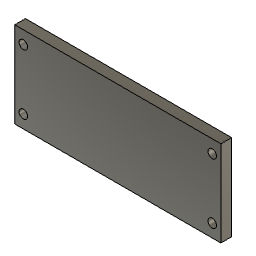
cementform_Wmiddle_80x40_plateB (Autodesk Fusion 360 design; units mm, degrees)
Autodesk Fusion 360 part; units mm, degrees
sketch "baseplate" plane through (0, 0, 0) normal (0, 1, 0) x (1, 0, 0)
  line L0 (0, 0) -> (80, 0)
  line L1 (80, 0) -> (80, -40)
  line L2 (80, -40) -> (0, -40)
  line L3 (0, -40) -> (0, 0)
  dimension "d1" = 80
  dimension "d2" = 40
  constraint horizontal L0
  constraint vertical L1
  constraint horizontal L2
  constraint vertical L3
  constraint coincident L0.start L3.end
  measures "d1" distance of L0.start L0.end
  measures "d2" distance of L0.start L2.end
sketch "pryamid_base" plane through (0, 0, 0) normal (0, 1, 0) x (1, 0, 0)
  line L0 (5, -35) -> (15, -35)
  line L1 (15, -35) -> (15, -25)
  line L2 (15, -25) -> (5, -25)
  line L3 (5, -25) -> (5, -35)
  line L4 (35, -35) -> (35, -25)
  line L5 (35, -25) -> (25, -25)
  line L6 (25, -35) -> (35, -35)
  line L7 (25, -25) -> (25, -35)
  line L8 (75, -35) -> (75, -25)
  line L9 (45, -35) -> (55, -35)
  line L10 (55, -25) -> (45, -25)
  line L11 (65, -25) -> (65, -35)
  line L12 (65, -35) -> (75, -35)
  line L13 (55, -35) -> (55, -25)
  line L14 (45, -25) -> (45, -35)
  line L15 (75, -25) -> (65, -25)
  line L16 (35, -5) -> (25, -5)
  line L17 (35, -15) -> (35, -5)
  line L18 (15, -5) -> (5, -5)
  line L19 (25, -5) -> (25, -15)
  line L20 (45, -15) -> (55, -15)
  line L21 (55, -15) -> (55, -5)
  line L22 (5, -5) -> (5, -15)
  line L23 (45, -5) -> (45, -15)
  line L24 (75, -15) -> (75, -5)
  line L25 (65, -5) -> (65, -15)
  line L26 (75, -5) -> (65, -5)
  line L27 (55, -5) -> (45, -5)
  line L28 (65, -15) -> (75, -15)
  line L29 (5, -15) -> (15, -15)
  line L30 (15, -15) -> (15, -5)
  line L31 (25, -15) -> (35, -15)
  dimension "d3" = 10
  dimension "d4" = 10
  dimension "d5" = 10
  dimension "d6" = 10
  dimension "d7" = 10
  dimension "d8" = 10
  dimension "d9" = 10
  dimension "d10" = 10
  dimension "d11" = 10
  dimension "d12" = 10
  dimension "d13" = 10
  dimension "d14" = 10
  dimension "d15" = 10
  dimension "d16" = 10
  dimension "d17" = 10
  dimension "d18" = 10
  constraint horizontal L0
  constraint vertical L1
  constraint horizontal L2
  constraint vertical L3
  constraint horizontal L6
  constraint vertical L4
  constraint horizontal L5
  constraint vertical L7
  constraint horizontal L9
  constraint vertical L13
  constraint horizontal L10
  constraint vertical L14
  constraint horizontal L12
  constraint vertical L8
  constraint horizontal L15
  constraint vertical L11
  constraint horizontal L29
  constraint vertical L30
  constraint horizontal L18
  constraint vertical L22
  constraint horizontal L31
  constraint vertical L17
  constraint horizontal L16
  constraint vertical L19
  constraint horizontal L20
  constraint vertical L21
  constraint horizontal L27
  constraint vertical L23
  constraint horizontal L28
  constraint vertical L24
  constraint horizontal L26
  constraint vertical L25
  measures "d3" distance of L0.start L0.end
  measures "d4" distance of L0.start L2.end
  measures "d5" distance of L6.start L4.start
  measures "d6" distance of L6.start L5.end
  measures "d7" distance of L9.start L9.end
  measures "d8" distance of L9.start L10.end
  measures "d9" distance of L8.start L11.end
  measures "d10" distance of L11.start L11.end
  measures "d11" distance of L22.end L29.end
  measures "d12" distance of L22.end L18.end
  measures "d13" distance of L17.start L19.end
  measures "d14" distance of L16.end L19.end
  measures "d15" distance of L20.start L20.end
  measures "d16" distance of L20.start L23.start
  measures "d17" distance of L24.start L25.end
  measures "d18" distance of L25.start L25.end
ref_plane "WorkPlane1" through (0, 4.5, 0) normal (0, 1, 0) x (0, 0, 1)
sketch "pryamid_offsetplane" plane through (0, 4.5, 0) normal (0, 1, 0) x (1, 0, 0)
  line L0 (7.5, -32.5) -> (12.5, -32.5)
  line L1 (12.5, -32.5) -> (12.5, -27.5)
  line L2 (12.5, -27.5) -> (7.5, -27.5)
  line L3 (7.5, -27.5) -> (7.5, -32.5)
  line L4 (27.5, -27.5) -> (27.5, -32.5)
  line L5 (32.5, -32.5) -> (32.5, -27.5)
  line L6 (27.5, -32.5) -> (32.5, -32.5)
  line L7 (32.5, -27.5) -> (27.5, -27.5)
  line L8 (7.5, -27.5) -> (7.5, -32.5)
  line L9 (12.5, -32.5) -> (12.5, -27.5)
  line L10 (7.5, -32.5) -> (12.5, -32.5)
  line L11 (12.5, -27.5) -> (7.5, -27.5)
  line L12 (47.5, -27.5) -> (47.5, -32.5)
  line L13 (52.5, -32.5) -> (52.5, -27.5)
  line L14 (47.5, -32.5) -> (52.5, -32.5)
  line L15 (52.5, -27.5) -> (47.5, -27.5)
  line L16 (67.5, -27.5) -> (67.5, -32.5)
  line L17 (72.5, -32.5) -> (72.5, -27.5)
  line L18 (67.5, -32.5) -> (72.5, -32.5)
  line L19 (72.5, -27.5) -> (67.5, -27.5)
  line L20 (72.5, -12.5) -> (72.5, -7.5)
  line L21 (27.5, -7.5) -> (27.5, -12.5)
  line L22 (12.5, -12.5) -> (12.5, -7.5)
  line L23 (72.5, -7.5) -> (67.5, -7.5)
  line L24 (12.5, -7.5) -> (7.5, -7.5)
  line L25 (52.5, -12.5) -> (52.5, -7.5)
  line L26 (7.5, -7.5) -> (7.5, -12.5)
  line L27 (7.5, -12.5) -> (12.5, -12.5)
  line L28 (47.5, -12.5) -> (52.5, -12.5)
  line L29 (67.5, -7.5) -> (67.5, -12.5)
  line L30 (47.5, -7.5) -> (47.5, -12.5)
  line L31 (67.5, -12.5) -> (72.5, -12.5)
  line L32 (32.5, -7.5) -> (27.5, -7.5)
  line L33 (52.5, -7.5) -> (47.5, -7.5)
  line L34 (27.5, -12.5) -> (32.5, -12.5)
  line L35 (12.5, -7.5) -> (7.5, -7.5)
  line L36 (32.5, -12.5) -> (32.5, -7.5)
  line L37 (12.5, -12.5) -> (12.5, -7.5)
  line L38 (7.5, -12.5) -> (12.5, -12.5)
  line L39 (7.5, -7.5) -> (7.5, -12.5)
  constraint vertical L1
  constraint horizontal L2
  constraint vertical L5
  constraint horizontal L7
  constraint vertical L9
  constraint horizontal L11
  constraint vertical L13
  constraint horizontal L15
  constraint vertical L17
  constraint horizontal L19
  constraint vertical L37
  constraint horizontal L35
  constraint vertical L36
  constraint horizontal L32
  constraint vertical L22
  constraint horizontal L24
  constraint vertical L25
  constraint horizontal L33
  constraint vertical L20
  constraint horizontal L23
extrude "Extrude1" add sketch "baseplate" against normal blind 5
loft "Loft1" add profiles "pryamid_base", "pryamid_offsetplane" section 1 contours L0 L1 L2 L3 section 2 contours L0 L1 L2 L3 L8 L9 L10 L11
loft "Loft2" add profiles "pryamid_base", "pryamid_offsetplane" section 1 contours L4 L5 L6 L7 section 2 contours L4 L5 L6 L7
loft "Loft3" add profiles "pryamid_base", "pryamid_offsetplane" section 1 contours L9 L10 L13 L14 section 2 contours L12 L13 L14 L15
loft "Loft4" add profiles "pryamid_base", "pryamid_offsetplane" section 1 contours L8 L11 L12 L15 section 2 contours L16 L17 L18 L19
loft "Loft5" add profiles "pryamid_base", "pryamid_offsetplane" section 1 contours L24 L25 L26 L28 section 2 contours L20 L23 L29 L31
loft "Loft6" add profiles "pryamid_base", "pryamid_offsetplane" section 1 contours L20 L21 L23 L27 section 2 contours L25 L28 L30 L33
loft "Loft7" add profiles "pryamid_base", "pryamid_offsetplane" section 1 contours L16 L17 L19 L31 section 2 contours L21 L32 L34 L36
loft "Loft8" add profiles "pryamid_base", "pryamid_offsetplane" section 1 contours L18 L22 L29 L30 section 2 contours L22 L24 L26 L27 L35 L37 L38 L39
sketch "sidewall" plane through (0, 0, 0) normal (0, 1, 0) x (1, 0, 0)
  line L0 (0, 0) -> (-8, 0)
  line L1 (-8, 0) -> (-8, -40)
  line L2 (-8, -40) -> (0, -40)
  line L3 (0, -40) -> (0, 0)
  dimension "d22" = 8
  constraint horizontal L0
  constraint vertical L1
  constraint horizontal L2
  constraint vertical L3
  constraint coincident L0.start L3.end
  measures "d22" distance of L1.end L2.end
extrude "Extrude2" add sketch "sidewall" along normal blind 0 and the other way blind 5
sketch "sidemount" plane through (0, 0, 0) normal (0, 1, 0) x (1, 0, 0)
  line L0 (80, 0) -> (88, 0)
  line L1 (88, 0) -> (88, -40)
  line L2 (88, -40) -> (80, -40)
  line L3 (80, -40) -> (80, 0)
  constraint horizontal L0
  constraint vertical L1
  constraint horizontal L2
  constraint vertical L3
extrude "Extrude3" add sketch "sidemount" against normal blind 5
sketch "holes" plane through (0, -5, 0) normal (0, -1, 0) x (1, 0, 0)
  line L0 (88, 40) -> (-8, 40)
  line L1 (-8, 40) -> (-8, 0)
  line L2 (-8, 0) -> (88, 0)
  line L3 (88, 0) -> (88, 40)
  line L4 (-8, 0) -> (-4, 0)
  line L5 (-8, 6) -> (-8, 0)
  line L6 (-4, 40) -> (-8, 40)
  line L7 (-8, 40) -> (-8, 34)
  circle A0 centre (-4, 34) radius 2
  circle A1 centre (-4, 6) radius 2
  circle A2 centre (-4, 34) radius 3.4
  circle A3 centre (-4, 6) radius 3.4
  dimension "d29" = 6
  dimension "d30" = 4
  dimension "d31" = 4
  dimension "d32" = 6.8
  dimension "d33" = 6.8
  constraint horizontal L4
  constraint vertical L5
  constraint coincident L1.end L2.start
  constraint horizontal L6
  constraint vertical L7
  constraint coincident L0 L6.start
  constraint concentric A0 A2
  constraint concentric A1 A3
  measures "d29" distance of L6.start A0.centre
  measures "d30" diameter of A0
  measures "d31" diameter of A1
  measures "d32" diameter of A2
  measures "d33" diameter of A3
extrude "Extrude4" cut sketch "holes" against normal blind 51 contours A0 | A1
sketch "Sketch7" plane through (0, -5, 0) normal (0, -1, 0) x (1, 0, 0)
  circle A0 centre (84, 34) radius 2
  circle A1 centre (84, 6) radius 2
  circle A2 centre (84, 34) radius 3.4
  circle A3 centre (84, 6) radius 3.4
  dimension "d42" = 4
  dimension "d43" = 4
  dimension "d44" = 6.8
  dimension "d45" = 6.8
  constraint concentric A0 A2
  constraint concentric A1 A3
  measures "d42" diameter of A0
  measures "d43" diameter of A1
  measures "d44" diameter of A2
  measures "d45" diameter of A3
extrude "Extrude6" cut sketch "Sketch7" against normal blind 16 contours A0 | A1
